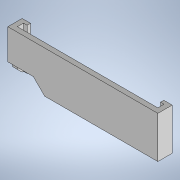
# Autodesk Inventor part: Крышка аккумулятора
Saved by Autodesk Inventor 2020 (Build 240168000, 168)
## iProperties
Created: 2021-04-26
Part Number: Крышка аккумулятора
Material: Типовые
Document SubType Name: Modeling
Designer: Антон
Density: 1 g/cm^3
Appearance: По умолчанию
Author: Антон
Autodesk Inventor part; units mm, degrees
ref_plane "YZ Plane" through (0, 0, 0) normal (1, 0, 0) x (0, 1, 0)
sketch "Эскиз1" plane through (0, 0, 0) normal (0, 0, 1) x (1, 0, 0)
  line L0 (0, 0) -> (62.9, 0)
  line L1 (62.9, 0) -> (62.9, 8)
  line L2 (62.9, 8) -> (0, 8)
  line L3 (0, 8) -> (0, 0)
  dimension "d0" = 62.9
  dimension "d1" = 8
  constraints: 8 end point, 2 parallel, 1 horizontal, 1 perpendicular
  measures "d0" distance of L2.end L1.end
  measures "d1" distance of L1.end L0.end
extrude "Выдавливание1" add sketch "Эскиз1" along normal blind 2
sketch "Эскиз2" plane through (0, 8, 0) normal (0, 1, 0) x (1, 0, 0)
  line L0 (0, 0) -> (2, 0)
  line L1 (2, 0) -> (2, 4)
  line L2 (2, 4) -> (0, 4)
  line L3 (0, 4) -> (0, 0)
  line L4 (2, 4) -> (3.5, 4)
  line L5 (3.5, 4) -> (3.5, 2.6)
  line L6 (3.5, 2.6) -> (2, 2.6)
  line L7 (2, 2.6) -> (2, 4)
  point P0 (2, 2.6)
  point P1 (2, 2.6)
  dimension "d4" = 2
  dimension "d5" = 4
  dimension "d6" = 1.5
  dimension "d7" = 1.4
  constraints: 16 end point, 4 parallel, 2 horizontal, 2 perpendicular
  measures "d4" distance of L2.end L1.end
  measures "d5" distance of L1.end L0.end
  measures "d6" distance of L5.end L6.end
  measures "d7" distance of L4.end L5.end
extrude "Выдавливание2" add sketch "Эскиз2" against normal up to surface (8 mm away)
ref_plane "РабПлоскость1" through (31.45, 0, 2) normal (-1, 0, 0) x (0, 0, 1)
mirror "Зеркальное отражение1" about plane through (31.45, 0, 2) normal (-1, 0, 0) of "Выдавливание2"
sketch "Эскиз6" plane through (0, 0, 2) normal (0, -1, 0) x (1, 0, 0)
  line L0 (62.9, -2) -> (10.7, -2)
  line L1 (10.7, -2) -> (10.7, 0)
  line L2 (10.7, 0) -> (62.9, 0)
  line L3 (62.9, 0) -> (62.9, -2)
  line L4 (2, -2) -> (60.9, -2) projected
  line L5 (0, 0) -> (62.9, 0) projected
  line L6 (2, -2) -> (60.9, -2) projected
  line L7 (60.9, -2) -> (60.9, -4.6) projected
  line L8 (60.9, -4.6) -> (59.4, -4.6) projected
  line L9 (59.4, -4.6) -> (59.4, -6) projected
  line L10 (59.4, -6) -> (62.9, -6) projected
  line L11 (62.9, -6) -> (62.9, 0) projected
  line L12 (0, 0) -> (62.9, 0) projected
  line L13 (0, -6) -> (0, 0) projected
  line L14 (3.5, -6) -> (0, -6) projected
  line L15 (3.5, -4.6) -> (3.5, -6) projected
  line L16 (2, -4.6) -> (3.5, -4.6) projected
  line L17 (2, -2) -> (2, -4.6) projected
  line L18 (60.9, -2) -> (62.9, -2)
  line L19 (2, -2) -> (0, -2)
  line L20 (62.9, -6) -> (62.9, 0) projected
  point P0 (0, -2)
  dimension "d29" = 10.7
  constraints: 12 end point, 3 collinear, 3 horizontal, 2 parallel, 1 perpendicular, 1 point on line
  measures "d29" distance between parallel lines of L13 L1
extrude "Выдавливание6" add sketch "Эскиз6" along normal blind 4.75 contours L11 L10 L9 L8 L7 L0 | L0 L1 L2 L3 | L17 L16 L15 L14 L13 L19
ref_plane "РабПлоскость2" through (0, 4, 2) normal (0, 1, 0) x (1, 0, 0)
sketch "Эскиз7" plane through (0, 8, 2) normal (0, 1, 0) x (1, 0, 0)
  line L0 (60.9, 2) -> (2, 2) projected
  line L1 (2, 2) -> (2, 4.6) projected
  line L2 (2, 4.6) -> (3.5, 4.6) projected
  line L3 (3.5, 4.6) -> (3.5, 6) projected
  line L4 (3.5, 6) -> (0, 6) projected
  line L5 (0, 6) -> (0, 0) projected
  line L6 (62.9, 0) -> (0, 0) projected
  line L7 (62.9, 6) -> (62.9, 0) projected
  line L8 (59.4, 6) -> (62.9, 6) projected
  line L9 (59.4, 4.6) -> (59.4, 6) projected
  line L10 (60.9, 4.6) -> (59.4, 4.6) projected
  line L11 (60.9, 2) -> (60.9, 4.6) projected
  point P0 (0, 2)
extrude "Выдавливание7" add sketch "Эскиз7" along normal blind 4.75
sketch "Эскиз5" plane through (0, 0, 2) normal (0, 0, 1) x (1, 0, 0)
  line L0 (49.7, 12.75) -> (47.2, 12.75)
  line L1 (47.2, 12.75) -> (47.2, 4.75)
  line L2 (47.2, 4.75) -> (49.7, 4.75)
  line L3 (49.7, 4.75) -> (49.7, 12.75)
  line L4 (62.9, 0) -> (62.9, 8) projected
  line L5 (62.9, 4) -> (49.7, 4)
  line L6 (0, 12.75) -> (62.9, 12.75) projected
  point P0 (0, 0)
  dimension "d15" = 2.5
  dimension "d16" = 8
  dimension "d19" = 13.2
  constraints: 10 end point, 2 horizontal, 2 parallel, 1 collinear, 1 midpoint, 1 perpendicular, 1 point on line
  measures "d15" distance of L2.end L1.end
  measures "d16" distance of L1.end L0.end
  measures "d19" distance of L5.start L5.end
extrude "Выдавливание5" [suppressed]
chamfer "Фаска1" distance 4.75 angle 45 1 edges at (10.7, -4.75, 1)
chamfer "Фаска2" distance 2 angle 45 1 edges at (1, -4.75, 0)
